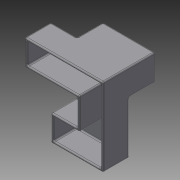
# Autodesk Inventor part: Piece 7
Saved by Autodesk Inventor 2014 (Build 180170000, 170)
## iProperties
Created: 2013-06-22
Part Number: Piece 7
Material: Generic
Document SubType Name: Modeling
Designer: ACooper
Mass: 2.36954 g
Surface Area: 47.3098 cm^2
Volume: 2.36954 cm^3
Density: 1 g/cm^3
Appearance: IM Dark Blue
Author: ACooper
Autodesk Inventor part; units mm, degrees
ref_plane "YZ Plane" through (0, 0, 0) normal (1, 0, 0) x (0, 1, 0)
ref_plane "XZ Plane" through (0, 0, 0) normal (0, 1, 0) x (-1, 0, 0)
ref_plane "XY Plane" through (0, 0, 0) normal (0, 0, 1) x (1, 0, 0)
derived "Cube Master.ipt"
sketch "Sketch1" plane through (0, 0, 0) normal (0, 0, 1) x (1, 0, 0)
  line L0 (0, 0) -> (10, 0)
  line L1 (10, 0) -> (10, 10)
  line L2 (10, 10) -> (0, 10)
  line L3 (0, 10) -> (0, 0)
  line L4 (0, 0) -> (10, 0)
  line L5 (10, 0) -> (10, -10)
  line L6 (10, -10) -> (0, -10)
  line L7 (0, -10) -> (0, 0)
  line L8 (0, 0) -> (-10, 0)
  line L9 (-10, 0) -> (-10, 10)
  line L10 (-10, 10) -> (0, 10)
  line L11 (0, 10) -> (0, 0)
  line L12 (0, 0) -> (-10, 0)
  line L13 (-10, 0) -> (-10, -10)
  line L14 (-10, -10) -> (0, -10)
  line L15 (0, -10) -> (0, 0)
  line L16 (0, 10) -> (10, 10)
  line L17 (10, 10) -> (10, 20)
  line L18 (10, 20) -> (0, 20)
  line L19 (0, 20) -> (0, 10)
  line L20 (10, 0) -> (20, 0)
  line L21 (20, 0) -> (20, 10)
  line L22 (20, 10) -> (10, 10)
  line L23 (10, 10) -> (10, 0)
  line L24 (10, 0) -> (20, 0)
  line L25 (20, 0) -> (20, -10)
  line L26 (20, -10) -> (10, -10)
  line L27 (10, -10) -> (10, 0)
  line L28 (0, -10) -> (10, -10)
  line L29 (10, -10) -> (10, -20)
  line L30 (10, -20) -> (0, -20)
  line L31 (0, -20) -> (0, -10)
  line L32 (0, -10) -> (-10, -10)
  line L33 (-10, -10) -> (-10, -20)
  line L34 (-10, -20) -> (0, -20)
  line L35 (0, -20) -> (0, -10)
  line L36 (-10, 0) -> (-20, 0)
  line L37 (-20, 0) -> (-20, -10)
  line L38 (-20, -10) -> (-10, -10)
  line L39 (-10, -10) -> (-10, 0)
  line L40 (-10, 0) -> (-20, 0)
  line L41 (-20, 0) -> (-20, 10)
  line L42 (-20, 10) -> (-10, 10)
  line L43 (-10, 10) -> (-10, 0)
  line L44 (0, 10) -> (-10, 10)
  line L45 (-10, 10) -> (-10, 20)
  line L46 (-10, 20) -> (0, 20)
  line L47 (0, 20) -> (0, 10)
  line L48 (10, 10) -> (20, 10)
  line L49 (20, 10) -> (20, 20)
  line L50 (20, 20) -> (10, 20)
  line L51 (10, 20) -> (10, 10)
  line L52 (10, -10) -> (20, -10)
  line L53 (20, -10) -> (20, -20)
  line L54 (20, -20) -> (10, -20)
  line L55 (10, -20) -> (10, -10)
  line L56 (-10, -10) -> (-20, -10)
  line L57 (-20, -10) -> (-20, -20)
  line L58 (-20, -20) -> (-10, -20)
  line L59 (-10, -20) -> (-10, -10)
  line L60 (-10, 10) -> (-20, 10)
  line L61 (-20, 10) -> (-20, 20)
  line L62 (-20, 20) -> (-10, 20)
  line L63 (-10, 20) -> (-10, 10)
ref_plane "Work Plane1" through (-10, 20, 0) normal (1, 0, 0) x (0, 1, 0)
ref_plane "Work Plane2" through (-20, 20, 0) normal (1, 0, 0) x (0, 1, 0)
ref_plane "Work Plane3" through (10, 20, 0) normal (1, 0, 0) x (0, 1, 0)
ref_plane "Work Plane4" through (20, 20, 0) normal (1, 0, 0) x (0, 1, 0)
ref_plane "Work Plane5" through (0, 0, 20) normal (0, 0, 1) x (1, 0, 0)
ref_plane "Work Plane6" through (0, 0, 10) normal (0, 0, 1) x (1, 0, 0)
ref_plane "Work Plane7" through (0, 0, -20) normal (0, 0, 1) x (1, 0, 0)
ref_plane "Work Plane8" through (0, 0, -10) normal (0, 0, 1) x (1, 0, 0)
extrude "Extrusion1" add sketch "Sketch1" against normal up to surface (10 mm away) from surface at 0 contours L0 L5 L6 L7 | L20 L25 L26 L5 | L1 L22 L21 L20 | L19 L18 L17 L2 | L10 L45 L46 L19 | L17 L50 L49 L22
extrude "Extrusion2" add sketch "Sketch1" against normal up to surface (20 mm away) from surface at 0 contours L19 L18 L17 L2 | L17 L50 L49 L22
shell "Shell1" thickness 1 removed faces 1 at (6.6667, 16.6667, 0)
fillet "Fillet1" radius 0.49 25 edges at (10, 0, -5) (10, 10, -5) (15, 10, -10) (0, 15, -10) (1, -1, -4.5) (6, -1, -9) (11, 5, -9) (1, -9, -4.5) (1, -5, -9) (19, 1, -9) (10, -9, -9) (19, 11, -14) (10, 11, -19) (1, 11, -14) (-4, 11, -9) (-9, 11, -4.5) (19, -9, -4.5) (19, 19, -9.5) (19, 15, -19) (-9, 19, -4.5) (-4, 19, -9) (1, 19, -14) (10, 19, -19) (1, 15, -19) (-9, 15, -9)
fillet "Fillet1" radius 0.49 41 edges at (0, 0, -5) (5, 0, 0) (5, 0, -10) (10, 5, 0) (10, 5, -10) (0, -10, -5) (0, -5, 0) (0, -5, -10) (20, 0, -10) (10, -10, -10) (0, 10, 0) (-10, 10, -5) (-5, 10, -10) (0, 10, -15) (10, 10, -20) (20, 10, -15) (20, -10, -5) (10, -10, 0) (20, 5, 0) (20, 15, -20) (20, 20, -10) (5, 20, 0) (10, 20, -20) (0, 20, -15) (-5, 20, -10) (-10, 20, -5) (0, 15, -20) (-10, 15, -10) (-10, 15, 0) (11, 5, 0) (1, 11, 0) (-9, 15, 0) (5, 19, 0) (19, 5, 0) (10, -9, 0) (1, -5, 0) (6, -1, 0) (11, -1, -4.5) (11, 11, -4.5) (15, 11, -9) (1, 15, -9)
equation "\"d6\" = ShellThickness"
equation "\"d7\" = Fillets"
equation "\"d8\" = Fillets"
equation "\"ShellThickness\" = 1"
equation "\"Fillets\" = 0.49"
body "Solid1"
